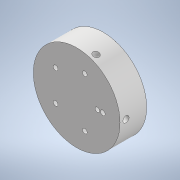
# Autodesk Inventor part: Vial upper holder
Saved by Autodesk Inventor 2022 (Build 260153000, 153)
## iProperties
Created: 2022-06-21
Part Number: Vial upper holder
Material: Generic
Document SubType Name: Modeling
Designer: efred
Density: 1 g/cm^3
Appearance: Default
Author: efred
Autodesk Inventor part; units mm, degrees
ref_plane "YZ Plane" through (0, 0, 0) normal (1, 0, 0) x (0, 1, 0)
ref_plane "XZ Plane" through (0, 0, 0) normal (0, 1, 0) x (-1, 0, 0)
ref_plane "XY Plane" through (0, 0, 0) normal (0, 0, 1) x (1, 0, 0)
sketch "Sketch1" plane through (0, 0, 0) normal (0, 0, 1) x (1, 0, 0)
  circle A0 centre (0.0008, 0.0003) radius 14.3992 projected
  line L0 (19.3992, 0) -> (-19.3992, 0) construction
  circle A1 centre (-29.3992, 0) radius 10
  circle A2 centre (-29.3992, 0) radius 48.7983
  circle A3 centre (0, 0) radius 14.4
  circle A4 centre (-20.3143, 27.9603) radius 14.4
  circle A5 centre (-53.1836, 17.2804) radius 14.4
  circle A6 centre (-53.1836, -17.2804) radius 14.4
  circle A7 centre (-20.3143, -27.9603) radius 14.4
  dimension "d2" = 20
  dimension "d0" = 28.7983
  dimension "d1" = 38.7983
  dimension "d5" = 360
  constraints: 5 centre point, 3 coincident, 3 horizontal alignment, 2 end point, 1 horizontal, 1 midpoint, 1 tangent, 15 other
  measures "d0" diameter of A0
  measures "d1" distance of L0.start L0.end
extrude "Extrusion1" add sketch "Sketch1" along normal blind 1 and the other way blind 9
ref_plane "Work Plane1" through (0, 0, 0) normal (0, 0, 1) x (1, 0, 0)
sketch "Sketch2" plane through (0, 0, 0) normal (0, 0, 1) x (1, 0, 0)
  circle A0 centre (0, 0) radius 10.75 projected
  circle A1 centre (0, 0) radius 14.4 projected
extrude "Extrusion2" add sketch "Sketch2" along normal up to surface (1 mm away)
pattern_circular "Circular Pattern1" count 5 over 360 about axis through (-29.3992, 0, 0) along (0, 0, 1) of "Extrusion2"
sketch "Sketch3" plane through (-29.3992, 0, 1) normal (0, 0, 1) x (1, 0, 0)
  line L0 (27.0833, -1.3) -> (25.5992, -1.3) construction
  line L1 (25.5992, -1.3) -> (25.5992, 1.3) construction
  line L2 (25.5992, 1.3) -> (27.0833, 1.3) construction
  line L3 (28.0992, 2.3159) -> (28.0992, 3.8) construction
  line L4 (28.0992, 3.8) -> (30.6992, 3.8) construction
  line L5 (30.6992, 3.8) -> (30.6992, 2.3159) construction
  line L6 (31.715, 1.3) -> (33.1992, 1.3) construction
  line L7 (33.1992, 1.3) -> (33.1992, -1.3) construction
  line L8 (33.1992, -1.3) -> (31.715, -1.3) construction
  line L9 (30.6992, -2.3159) -> (30.6992, -3.8) construction
  line L10 (30.6992, -3.8) -> (28.0992, -3.8) construction
  line L11 (28.0992, -3.8) -> (28.0992, -2.3159) construction
  circle A0 centre (29.3992, 0) radius 2.6558
  circle A1 centre (0, 0) radius 48.7983 projected
  circle A2 centre (9.0848, 27.9603) radius 2.6558
  circle A3 centre (-23.7844, 17.2804) radius 2.6558
  circle A4 centre (-23.7844, -17.2804) radius 2.6558
  circle A5 centre (9.0848, -27.9603) radius 2.6558
  arc A6 (31.715, 1.3) -> (30.6992, 2.3159) centre (29.3992, 0) ccw projected
  arc A7 (30.6992, -2.3159) -> (31.715, -1.3) centre (29.3992, 0) ccw projected
  arc A8 (27.0833, -1.3) -> (28.0992, -2.3159) centre (29.3992, 0) ccw projected
  arc A9 (28.0992, 2.3159) -> (27.0833, 1.3) centre (29.3992, 0) ccw projected
  arc A10 (30.8992, -4.7697) -> (34.1689, -1.5) centre (29.3992, 0) ccw projected
  line L12 (34.1689, -1.5) -> (41.8088, -1.5) projected
  arc A11 (30.8992, -12.4097) -> (41.8088, -1.5) centre (29.3992, 0) ccw projected
  line L13 (30.8992, -12.4097) -> (30.8992, -4.7697) projected
  line L14 (27.8992, -4.7697) -> (27.8992, -12.4097) projected
  arc A12 (16.9895, -1.5) -> (27.8992, -12.4097) centre (29.3992, 0) ccw projected
  line L15 (16.9895, -1.5) -> (24.6295, -1.5) projected
  line L16 (24.6295, 1.5) -> (16.9895, 1.5) projected
  arc A13 (27.8992, 12.4097) -> (16.9895, 1.5) centre (29.3992, 0) ccw projected
  line L17 (27.8992, 12.4097) -> (27.8992, 4.7697) projected
  line L18 (15.3337, -3.5231) -> (13.891, -4.4861) projected
  arc A14 (13.891, -4.4861) -> (13.6926, -5.0552) centre (14.1686, -4.902) ccw projected
  arc A15 (13.6926, -5.0552) -> (14.1178, -6.2235) centre (29.3992, 0) ccw projected
  arc A16 (14.1178, -6.2235) -> (14.6356, -6.5319) centre (14.5809, -6.0349) ccw projected
  line L19 (14.6356, -6.5319) -> (16.3598, -6.3422) projected
  arc A17 (16.3598, -6.3422) -> (17.3869, -8.1213) centre (29.3992, 0) ccw projected
  line L20 (17.3869, -8.1213) -> (16.3606, -9.5197) projected
  arc A18 (16.3606, -9.5197) -> (16.3688, -10.1223) centre (16.7637, -9.8155) ccw projected
  arc A19 (16.3688, -10.1223) -> (17.168, -11.0746) centre (29.3992, 0) ccw projected
  arc A20 (17.168, -11.0746) -> (17.76, -11.1874) centre (17.5386, -10.7391) ccw projected
  line L21 (17.76, -11.1874) -> (19.3153, -10.4195) projected
  arc A21 (19.3153, -10.4195) -> (20.889, -11.74) centre (29.3992, 0) ccw projected
  line L22 (20.889, -11.74) -> (20.4029, -13.405) projected
  arc A22 (20.4029, -13.405) -> (20.6167, -13.9685) centre (20.8828, -13.5452) ccw projected
  arc A23 (20.6167, -13.9685) -> (21.6934, -14.5901) centre (29.3992, 0) ccw projected
  arc A24 (21.6934, -14.5901) -> (22.2882, -14.4935) centre (21.9269, -14.148) ccw projected
  line L23 (22.2882, -14.4935) -> (23.4871, -13.24) projected
  arc A25 (23.4871, -13.24) -> (25.4176, -13.9426) centre (29.3992, 0) ccw projected
  line L24 (25.4176, -13.9426) -> (25.5302, -15.6735) projected
  arc A26 (25.5302, -15.6735) -> (25.9238, -16.1299) centre (26.0291, -15.6411) ccw projected
  arc A27 (25.9238, -16.1299) -> (27.1482, -16.3457) centre (29.3992, 0) ccw projected
  arc A28 (27.1482, -16.3457) -> (27.6741, -16.0516) centre (27.2164, -15.8504) ccw projected
  line L25 (27.6741, -16.0516) -> (28.372, -14.4636) projected
  arc A29 (28.372, -14.4636) -> (30.4263, -14.4636) centre (29.3992, 0) ccw projected
  line L26 (30.4263, -14.4636) -> (31.1242, -16.0516) projected
  arc A30 (31.1242, -16.0516) -> (31.6502, -16.3457) centre (31.5819, -15.8504) ccw projected
  arc A31 (31.6502, -16.3457) -> (32.8745, -16.1299) centre (29.3992, 0) ccw projected
  arc A32 (32.8745, -16.1299) -> (33.2681, -15.6735) centre (32.7692, -15.6411) ccw projected
  line L27 (33.2681, -15.6735) -> (33.3808, -13.9426) projected
  arc A33 (33.3808, -13.9426) -> (35.3112, -13.24) centre (29.3992, 0) ccw projected
  line L28 (35.3112, -13.24) -> (36.5101, -14.4935) projected
  arc A34 (36.5101, -14.4935) -> (37.105, -14.5901) centre (36.8715, -14.148) ccw projected
  arc A35 (37.105, -14.5901) -> (38.1816, -13.9685) centre (29.3992, 0) ccw projected
  arc A36 (38.1816, -13.9685) -> (38.3955, -13.405) centre (37.9155, -13.5452) ccw projected
  line L29 (38.3955, -13.405) -> (37.9093, -11.74) projected
  arc A37 (37.9093, -11.74) -> (39.483, -10.4195) centre (29.3992, 0) ccw projected
  line L30 (39.483, -10.4195) -> (41.0384, -11.1874) projected
  arc A38 (41.0384, -11.1874) -> (41.6304, -11.0746) centre (41.2597, -10.7391) ccw projected
  arc A39 (41.6304, -11.0746) -> (42.4295, -10.1223) centre (29.3992, 0) ccw projected
  arc A40 (42.4295, -10.1223) -> (42.4377, -9.5197) centre (42.0346, -9.8155) ccw projected
  line L31 (42.4377, -9.5197) -> (41.4114, -8.1213) projected
  arc A41 (41.4114, -8.1213) -> (42.4386, -6.3422) centre (29.3992, 0) ccw projected
  line L32 (42.4386, -6.3422) -> (44.1627, -6.5319) projected
  arc A42 (44.1627, -6.5319) -> (44.6805, -6.2235) centre (44.2174, -6.0349) ccw projected
  arc A43 (44.6805, -6.2235) -> (45.1057, -5.0552) centre (29.3992, 0) ccw projected
  arc A44 (45.1057, -5.0552) -> (44.9073, -4.4861) centre (44.6297, -4.902) ccw projected
  line L33 (44.9073, -4.4861) -> (43.4646, -3.5231) projected
  arc A45 (43.4646, -3.5231) -> (43.8214, -1.5) centre (29.3992, 0) ccw projected
  line L34 (43.8214, -1.5) -> (45.5064, -1.0885) projected
  arc A46 (45.5064, -1.0885) -> (45.8874, -0.6216) centre (45.3878, -0.6028) ccw projected
  arc A47 (45.8874, -0.6216) -> (45.8874, 0.6216) centre (29.3992, 0) ccw projected
  arc A48 (45.8874, 0.6216) -> (45.5064, 1.0885) centre (45.3878, 0.6028) ccw projected
  line L35 (45.5064, 1.0885) -> (43.8214, 1.5) projected
  arc A49 (43.8214, 1.5) -> (43.4646, 3.5231) centre (29.3992, 0) ccw projected
  line L36 (43.4646, 3.5231) -> (44.9073, 4.4861) projected
  arc A50 (44.9073, 4.4861) -> (45.1057, 5.0552) centre (44.6297, 4.902) ccw projected
  arc A51 (45.1057, 5.0552) -> (44.6805, 6.2235) centre (29.3992, 0) ccw projected
  arc A52 (44.6805, 6.2235) -> (44.1627, 6.5319) centre (44.2174, 6.0349) ccw projected
  line L37 (44.1627, 6.5319) -> (42.4386, 6.3422) projected
  arc A53 (42.4386, 6.3422) -> (41.4114, 8.1213) centre (29.3992, 0) ccw projected
  line L38 (41.4114, 8.1213) -> (42.4377, 9.5197) projected
  arc A54 (42.4377, 9.5197) -> (42.4295, 10.1223) centre (42.0346, 9.8155) ccw projected
  arc A55 (42.4295, 10.1223) -> (41.6304, 11.0746) centre (29.3992, 0) ccw projected
  arc A56 (41.6304, 11.0746) -> (41.0384, 11.1874) centre (41.2597, 10.7391) ccw projected
  line L39 (41.0384, 11.1874) -> (39.483, 10.4195) projected
  arc A57 (39.483, 10.4195) -> (37.9093, 11.74) centre (29.3992, 0) ccw projected
  line L40 (37.9093, 11.74) -> (38.3955, 13.405) projected
  arc A58 (38.3955, 13.405) -> (38.1816, 13.9685) centre (37.9155, 13.5452) ccw projected
  arc A59 (38.1816, 13.9685) -> (37.105, 14.5901) centre (29.3992, 0) ccw projected
  arc A60 (37.105, 14.5901) -> (36.5101, 14.4935) centre (36.8715, 14.148) ccw projected
  line L41 (36.5101, 14.4935) -> (35.3112, 13.24) projected
  arc A61 (35.3112, 13.24) -> (33.3808, 13.9426) centre (29.3992, 0) ccw projected
  line L42 (33.3808, 13.9426) -> (33.2681, 15.6735) projected
  arc A62 (33.2681, 15.6735) -> (32.8745, 16.1299) centre (32.7692, 15.6411) ccw projected
  arc A63 (32.8745, 16.1299) -> (31.6502, 16.3457) centre (29.3992, 0) ccw projected
  arc A64 (31.6502, 16.3457) -> (31.1242, 16.0516) centre (31.5819, 15.8504) ccw projected
  line L43 (31.1242, 16.0516) -> (30.4263, 14.4636) projected
  arc A65 (30.4263, 14.4636) -> (28.372, 14.4636) centre (29.3992, 0) ccw projected
  line L44 (28.372, 14.4636) -> (27.6741, 16.0516) projected
  arc A66 (27.6741, 16.0516) -> (27.1482, 16.3457) centre (27.2164, 15.8504) ccw projected
  arc A67 (27.1482, 16.3457) -> (25.9238, 16.1299) centre (29.3992, 0) ccw projected
  arc A68 (25.9238, 16.1299) -> (25.5302, 15.6735) centre (26.0291, 15.6411) ccw projected
  line L45 (25.5302, 15.6735) -> (25.4176, 13.9426) projected
  arc A69 (25.4176, 13.9426) -> (23.4871, 13.24) centre (29.3992, 0) ccw projected
  line L46 (23.4871, 13.24) -> (22.2882, 14.4935) projected
  arc A70 (22.2882, 14.4935) -> (21.6934, 14.5901) centre (21.9269, 14.148) ccw projected
  arc A71 (21.6934, 14.5901) -> (20.6167, 13.9685) centre (29.3992, 0) ccw projected
  arc A72 (20.6167, 13.9685) -> (20.4029, 13.405) centre (20.8828, 13.5452) ccw projected
  line L47 (20.4029, 13.405) -> (20.889, 11.74) projected
  arc A73 (20.889, 11.74) -> (19.3153, 10.4195) centre (29.3992, 0) ccw projected
  line L48 (19.3153, 10.4195) -> (17.76, 11.1874) projected
  arc A74 (17.76, 11.1874) -> (17.168, 11.0746) centre (17.5386, 10.7391) ccw projected
  arc A75 (17.168, 11.0746) -> (16.3688, 10.1223) centre (29.3992, 0) ccw projected
  arc A76 (16.3688, 10.1223) -> (16.3606, 9.5197) centre (16.7637, 9.8155) ccw projected
  line L49 (16.3606, 9.5197) -> (17.3869, 8.1213) projected
  arc A77 (17.3869, 8.1213) -> (16.3598, 6.3422) centre (29.3992, 0) ccw projected
  line L50 (16.3598, 6.3422) -> (14.6356, 6.5319) projected
  arc A78 (14.6356, 6.5319) -> (14.1178, 6.2235) centre (14.5809, 6.0349) ccw projected
  arc A79 (14.1178, 6.2235) -> (13.6926, 5.0552) centre (29.3992, 0) ccw projected
  arc A80 (13.6926, 5.0552) -> (13.891, 4.4861) centre (14.1686, 4.902) ccw projected
  line L51 (13.891, 4.4861) -> (15.3337, 3.5231) projected
  arc A81 (15.3337, 3.5231) -> (14.977, 1.5) centre (29.3992, 0) ccw projected
  arc A82 (14.977, -1.5) -> (15.3337, -3.5231) centre (29.3992, 0) ccw projected
  line L52 (30.8992, 4.7697) -> (30.8992, 12.4097) projected
  arc A83 (41.8088, 1.5) -> (30.8992, 12.4097) centre (29.3992, 0) ccw projected
  line L53 (41.8088, 1.5) -> (34.1689, 1.5) projected
  arc A84 (34.1689, 1.5) -> (30.8992, 4.7697) centre (29.3992, 0) ccw projected
  arc A85 (24.6295, -1.5) -> (27.8992, -4.7697) centre (29.3992, 0) ccw projected
  arc A86 (27.8992, 4.7697) -> (24.6295, 1.5) centre (29.3992, 0) ccw projected
  line L54 (14.977, 1.5) -> (14.977, -1.5) projected
  point P0 (29.3992, 0)
  point P1 (27.0992, -1.3279)
  point P2 (27.0992, 1.3279)
  point P3 (28.0713, 2.3)
  point P4 (30.7271, 2.3)
  point P5 (31.6992, 1.3279)
  point P6 (31.6992, -1.3279)
  point P7 (30.7271, -2.3)
  point P8 (28.0713, -2.3)
  point P9 (7.3078, 29.9339)
  point P10 (-26.2106, 16.2002)
  point P11 (-23.5068, -19.9217)
  point P12 (11.6826, -28.5124)
  point P13 (29.3992, 0)
  point P14 (29.3992, 0)
  point P15 (29.3992, 0)
  point P16 (29.3992, 0)
  point P17 (29.3992, 0)
  point P18 (29.3992, 0)
  point P19 (29.3992, 0)
  point P20 (29.3992, 0)
  point P21 (29.3992, 0)
  point P22 (29.3992, 0)
  point P23 (29.3992, 0)
  point P24 (29.3992, 0)
  point P25 (29.3992, 0)
  point P26 (29.3992, 0)
  point P27 (29.3992, 0)
  point P28 (29.3992, 0)
  point P29 (29.3992, 0)
  point P30 (29.3992, 0)
  point P31 (29.3992, 0)
  point P32 (29.3992, 0)
  point P33 (29.3992, 0)
  dimension "d18" = 360
  constraints: 31 other
extrude "Extrusion3" add sketch "Sketch3" along normal blind 20 contours A1 | A10 L12 A11 L13 | L14 A12 L15 A85 | L16 A13 L17 A86 | A82 L54 A81 L51 A80 A79 A78 L50 A77 L49 A76 A75 A74 L48 A73 L47 A72 A71 A70 L46 A69 L45 A68 A67 A66 L44 A65 L43 A64 A63 A62 L42 A61 L41 A60 A59 A58 L40 A57 L39 A56 A55 A54 L38 A53 L37 A52 A51 A50 L36 A49 L35 A48 A47 A46 L34 A45 L33 A44 A43 A42 L32 A41 L31 A40 A39 A38 L30 A37 L29 A36 A35 A34 L28 A33 L27 A32 A31 A30 L26 A29 L25 A28 A27 A26 L24 A25 L23 A24 A23 A22 L22 A21 L21 A20 A19 A18 L20 A17 L19 A16 A15 A14 L18 | L52 A83 L53 A84
sketch "Sketch4" plane through (0, 0, 0) normal (0, 1, 0) x (-1, 0, 0)
  line L0 (-19.3992, -9) -> (-19.3992, 21) projected
  circle A0 centre (-19.3992, 1) radius 16.7434 construction
  line L1 (10.75, 1) -> (-10.75, 1) construction
  circle A1 centre (-19.3992, 1) radius 9.7434 construction
  line L2 (-2.6558, 21) -> (-2.6558, 1) construction
  circle A2 centre (-19.3992, 1) radius 13.2434
  point P0 (0, 0)
  dimension "d22" = 7
  dimension "d23" = 3.5
  constraints: 3 centre point, 1 coincident, 1 line through centre, 1 point on line, 1 tangent
  measures "d22" radial gap between concentric circles of A0 A1
  measures "d23" radial gap between concentric circles of A1 A2
sketch "Sketch5" plane through (0, 0, 1) normal (0, 0, -1) x (-1, 0, 0)
  line L0 (-6.1558, 0) -> (-32.6425, 0) projected
  circle A0 centre (-6.1558, 0) radius 3.5
  circle A1 centre (0, 0) radius 2.6558 projected
  point P0 (0, 0)
  constraints: 1 centre point, 1 coincident, 1 tangent
sweep "Sweep1" cut profiles "Sketch5" path "Sketch4" path curves A2 contours A0
pattern_circular "Circular Pattern2" count 5 over 360 about axis through (-29.3992, 0, 0) along (0, 0, 1) of "Sweep1"
sketch "Sketch6" plane through (0, 0, 1) normal (0, 0, -1) x (-1, 0, 0)
  circle A0 centre (-6.1558, 0) radius 3.5 projected
  circle A1 centre (0, 0) radius 2.6558 projected
  circle A2 centre (0, 0) radius 2.6558 projected
  line L0 (0, 0) -> (0, 2.6558)
  circle A3 centre (6.1558, 0) radius 3.5 construction
  circle A4 centre (6.1558, 0) radius 2.5
  point P0 (0, 0)
  point P1 (-2.6558, 0)
  dimension "d13" = 5
  dimension "d14" = 360
  dimension "d29" = 5
  constraints: 2 centre point, 2 end point, 2 horizontal alignment, 1 coincident, 1 point on circle, 1 symmetric about line, 1 vertical, 1 other
  measures "d29" diameter of A4
extrude "Extrusion4" [suppressed]
pattern_circular "Circular Pattern3" [suppressed]
body "Solid1"
